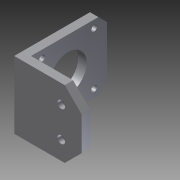
# Autodesk Inventor part: 13_0204_058
Saved by Autodesk Inventor 2012 SP1 (Build 160190100, 190)
## iProperties
Created: 2013-04-15
Part Number: 13_0204_058
Material: Default
Document SubType Name: Modeling
Designer: vogel
Density: 1 g/cm^3
Author: vogel
Autodesk Inventor part; units mm, degrees
ref_plane "YZ Plane" through (0, 0, 0) normal (1, 0, 0) x (0, 1, 0)
ref_plane "XZ Plane" through (0, 0, 0) normal (0, 1, 0) x (-1, 0, 0)
ref_plane "XY Plane" through (0, 0, 0) normal (0, 0, 1) x (1, 0, 0)
sketch "Skizze1" plane through (0, 0, 0) normal (0, 0, 1) x (1, 0, 0)
  line L0 (0, 0) -> (40, 0)
  line L1 (5, 5) -> (5, 50)
  line L2 (5, 50) -> (0, 50)
  line L3 (0, 50) -> (0, 0)
  line L4 (5, 5) -> (40, 5)
  line L5 (40, 5) -> (40, 0)
  line L6 (-8, 0) -> (48, 0) projected
  line L7 (0, -10) -> (0, 60) projected
  dimension "d0" = 50
  dimension "d3" = 40
  dimension "d4" = 5
  constraints: 12 end point, 3 perpendicular, 2 horizontal, 2 parallel
  measures "d0" distance of L2.end L0.start
  measures "d3" distance of L0.start L0.end
  measures "d4" distance of L1.end L2.end
extrude "Extrusion1" add sketch "Skizze1" along normal blind 40
sketch "Skizze2" plane through (0, 0, 0) normal (-1, 0, 0) x (0, 0, 1)
  line L0 (0, 50) -> (40, 50) projected
  line L1 (0, 0) -> (40, 0) projected
  line L2 (20, 50) -> (20, 0)
  point P0 (20, 27)
  dimension "d7" = 27
  constraints: 2 end point, 2 midpoint, 1 point on line
  measures "d7" distance from line of point (20, 27) L1
hole "Bohrung1" at (0, 27, 20) direction (1, 0, 0) diameter 22 end through all
sketch "Skizze4" plane through (0, 0, 0) normal (0, -1, 0) x (1, 0, 0)
  line L0 (40, 40) -> (0, 40) projected
  line L1 (0, 0) -> (0, 40) projected
  line L2 (0, 0) -> (40, 0) projected
  line L3 (40, 0) -> (40, 40) projected
  line L4 (28, 40) -> (28, 0)
  line L5 (0, 20) -> (40, 20)
  point P0 (28, 29)
  point P1 (28, 11)
  dimension "d24" = 12
  dimension "d25" = 18
  constraints: 4 end point, 4 point on line, 2 midpoint, 1 perpendicular, 1 symmetric about line
  measures "d24" distance between parallel lines of L3 L4
  measures "d25" distance of point (28, 29) point (28, 11)
hole "Bohrung3" at (28, 0, 29) at (28, 0, 11) direction (0, 1, 0) diameter 4.5 end through all
hole "Bohrung4" at (28, 5, 29) direction (0, -1, 0) diameter 4.5 end through all countersink diameter 9.2 countersink angle 90
hole "Bohrung5" at (28, 5, 11) direction (0, -1, 0) diameter 4.5 end through all countersink diameter 9.2 countersink angle 90
chamfer "Fase1" distance 10 angle 45 2 edges at (40, 2.5, 0) (40, 2.5, 40)
sketch "Skizze6" plane through (5, 5, 0) normal (1, 0, 0) x (0, 0, -1)
  circle A0 centre (-20, 22) radius 11 projected
  line L0 (0, 45) -> (-40, 45) projected
  line L1 (-20, 22) -> (-5.2877, 22)
  line L2 (0, -15.2) -> (0, 56.2) projected
  line L3 (8, -5) -> (-48, -5) projected
  line L4 (-20, 22) -> (-20, 10.2851)
  line L5 (-35.5, 37.5) -> (-4.5, 37.5)
  line L6 (-4.5, 37.5) -> (-4.5, 6.5)
  line L7 (-4.5, 6.5) -> (-35.5, 6.5)
  line L8 (-35.5, 6.5) -> (-35.5, 37.5)
  point P0 (0, -5)
  dimension "d54" = 31
  constraints: 12 end point, 4 coincident, 3 parallel, 3 perpendicular, 1 horizontal, 2 other
  measures "d54" distance of L5.start L5.end
hole "Bohrung6" at (5, 42.5, 35.5) at (5, 42.5, 4.5) at (5, 11.5, 4.5) at (5, 11.5, 35.5) direction (-1, 0, 0) diameter 3.4 end through all
chamfer "Fase2" distance 5 angle 45 2 edges at (2.5, 50, 40) (2.5, 50, 0)
